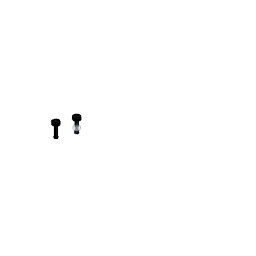
Buttons (Autodesk Fusion 360 design; units mm, degrees)
Autodesk Fusion 360 part; units mm, degrees
note: some values were not read from the file. Chosen so that the rebuilt part matches the saved one: a side. Set by a fixed rule: which sketch regions a step uses.
sketch "Sketch1" plane through (0, 0, 3.4) normal (0, 0, 1) x (0, 1, 0)
  line L0 (-23.4198, 1.314) -> (-23.4198, 6.814) construction
  arc A0 (-23.4198, 6.814) -> (-23.6698, 7.064) centre (-23.6698, 6.814) ccw construction
  line L1 (-23.6698, 7.064) -> (-29.1698, 7.064) construction
  arc A1 (-29.1698, 7.064) -> (-29.4198, 6.814) centre (-29.1698, 6.814) ccw construction
  line L2 (-29.4198, 6.814) -> (-29.4198, 1.314) construction
  arc A2 (-29.4198, 1.314) -> (-29.1698, 1.064) centre (-29.1698, 1.314) ccw construction
  line L3 (-29.1698, 1.064) -> (-23.6698, 1.064) construction
  arc A3 (-23.6698, 1.064) -> (-23.4198, 1.314) centre (-23.6698, 1.314) ccw construction
  circle A4 centre (-24.1698, 6.314) radius 0.5 construction
  circle A5 centre (-24.1698, 1.814) radius 0.5 construction
  circle A6 centre (-26.4198, 4.064) radius 1.8 construction
  circle A7 centre (-28.6698, 1.814) radius 0.5 construction
  circle A8 centre (-28.6698, 6.314) radius 0.5 construction
  line L4 (-48.8198, 1.314) -> (-48.8198, 6.814) construction
  arc A9 (-48.8198, 6.814) -> (-49.0698, 7.064) centre (-49.0698, 6.814) ccw construction
  line L5 (-49.0698, 7.064) -> (-54.5698, 7.064) construction
  arc A10 (-54.5698, 7.064) -> (-54.8198, 6.814) centre (-54.5698, 6.814) ccw construction
  line L6 (-54.8198, 6.814) -> (-54.8198, 1.314) construction
  arc A11 (-54.8198, 1.314) -> (-54.5698, 1.064) centre (-54.5698, 1.314) ccw construction
  line L7 (-54.5698, 1.064) -> (-49.0698, 1.064) construction
  arc A12 (-49.0698, 1.064) -> (-48.8198, 1.314) centre (-49.0698, 1.314) ccw construction
  circle A13 centre (-49.5698, 6.314) radius 0.5 construction
  circle A14 centre (-49.5698, 1.814) radius 0.5 construction
  circle A15 centre (-51.8198, 4.064) radius 1.8 construction
  circle A16 centre (-54.0698, 1.814) radius 0.5 construction
  circle A17 centre (-54.0698, 6.314) radius 0.5 construction
  circle A18 centre (-26.4198, 4.064) radius 1.725
  circle A19 centre (-26.4198, 4.064) radius 5 construction
  circle A20 centre (-26.4198, 4.064) radius 2.5
  circle A21 centre (-26.4198, 4.064) radius 4.6
  dimension "d37" = 3.45
  dimension "d38" = 10
  dimension "d40" = 5
  dimension "d202" = -0.4
  constraint concentric A6 A18
  constraint concentric A6 A19
  constraint concentric A6 A20
  measures "d37" diameter of A18
  measures "d38" diameter of A19
  measures "d40" diameter of A20
extrude "Extrude4" add sketch "Sketch1" along normal up to surface (18.97 mm away) from surface at 1.5 contours A18 | A20 makes body 1
extrude "Extrude5" add sketch "Sketch1" against normal blind 2.5 from surface at 20.47 contours A21 bodies 1
extrude "Extrude6" add sketch "Sketch1" against normal up to surface (1 mm away) from surface at 1.5 contours A20 bodies 1
copy_body "CopyPasteBodies1" bodies 1 makes body 2
move_body "Move1" bodies 2 to x (1, 0, 0) y (0, 1, 0) z (0, 0, 1) at (4.064, 26.4198, -4.9)
equation "d202 = -2 * offset"
equation "offset = 0.2 mm"
